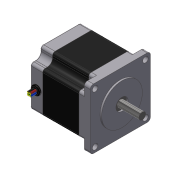
# Autodesk Inventor part: Motor Dummy
Saved by Autodesk Inventor 2015 (Build 190159000, 159)
## iProperties
Created: 2012-06-21
Part Number: Motor Dummy
Material: Generic
Document SubType Name: Modeling
Density: 4.80997 g/cm^3
Categories: <MemberInstance><Categories><Category DisplayName="" Mnemonic="CABLEANDHARNESS" InternalName="e4a7e005-5e42-4d16-b293-125e7f0d0512"><Category DisplayName="" Mnemonic="CONNECTORS" InternalName="6f634eba-a678-4820-a31d-2c2d5ee6728e"><CategoryParameter DisplayName="" Mnemonic="REFDES" InternalName="c3740e8c-60ab-4d5d-8584-52b73222f2f0"/><Category DisplayName="" Mnemonic="DISCRETEWIRE" InternalName="9a3407de-09b2-4cdb-8c40-9708d5144a28"/></Category></Category></Categories><FamilyTemplate><FamilyTemplateParameters></FamilyTemplateParameters></FamilyTemplate><CategoryParameterMap><ParamToTemplateMap><ParamToTemplate CategoryParameter="//CategoryParameter[@InternalName='c3740e8c-60ab-4d5d-8584-52b73222f2f0']" ConstantValue=""/></ParamToTemplateMap></CategoryParameterMap></MemberInstance>
Appearance: Glossy - Black
Mass: 1050 g
Surface Area: 350.377 cm^2
Volume: 218.297 cm^3
Autodesk Inventor part; units mm, degrees
ref_plane "YZ Plane" through (0, 0, 0) normal (1, 0, 0) x (0, 1, 0)
sketch "Sketch1" plane through (0, 0, 0) normal (1, 0, 0) x (0, 1, 0)
  line L0 (-28.2, 28.2) -> (28.2, 28.2)
  line L1 (28.2, 28.2) -> (28.2, -28.2)
  line L2 (28.2, -28.2) -> (-28.2, -28.2)
  line L3 (-28.2, -28.2) -> (-28.2, 28.2)
  point P0 (0, 0)
  point P1 (0, 28.2)
  point P2 (28.2, 0)
  dimension "d0" = 56.4
  dimension "d1" = 56.4
  constraints: 8 end point, 2 midpoint, 2 parallel, 1 horizontal, 1 horizontal alignment, 1 perpendicular, 1 vertical alignment
  measures "d0" distance of L0.start L0.end
  measures "d1" distance of L2.end L0.start
extrude "Extrusion1" add sketch "Sketch1" along normal mid plane 56
hole "Hole1" at (28, 0, 0) direction (-1, 0, 0) diameter 11.5 end through all
sketch "Sketch2" plane through (28, 0, 0) normal (1, 0, 0) x (0, 0, -1)
  line L0 (-23.57, -23.57) -> (23.57, -23.57) construction
  line L1 (23.57, -23.57) -> (23.57, 23.57) construction
  line L2 (23.57, 23.57) -> (-23.57, 23.57) construction
  line L3 (-23.57, 23.57) -> (-23.57, -23.57) construction
  point P0 (0, 0)
  point P1 (0, 23.57)
  point P2 (-23.57, 0)
  dimension "d13" = 47.14
  dimension "d15" = 47.14
  constraints: 8 end point, 4 coincident, 2 midpoint, 2 parallel, 1 horizontal, 1 horizontal alignment, 1 perpendicular, 1 vertical alignment
  measures "d13" distance of L1.end L2.end
  measures "d15" distance of L2.end L0.start
hole "Hole2" at (28, -23.57, 23.57) at (28, 23.57, 23.57) at (28, 23.57, -23.57) at (28, -23.57, -23.57) direction (-1, 0, 0) diameter 5.2 end through all
sketch "Sketch3" plane through (0, 0, 0) normal (0, 1, 0) x (-1, 0, 0)
  line L0 (-28, 28.2) -> (-28, -28.2) projected
  line L1 (73.9, 0) -> (-80.1, 0) projected
  line L2 (-28, 19.05) -> (-29.6, 19.05)
  line L3 (-29.6, 19.05) -> (-29.6, 3.175)
  line L4 (-29.6, 3.175) -> (-48.6, 3.175)
  line L5 (-48.6, 3.175) -> (-48.6, 0)
  line L6 (-28, 19.05) -> (-28, 0)
  line L7 (-29.6, 5.75) -> (-28, 5.75)
  line L8 (-28, 5.75) -> (25, 5.75)
  line L9 (25, 5.75) -> (25, 0)
  line L10 (25, 3.175) -> (42.4, 3.175)
  line L11 (42.4, 3.175) -> (42.4, 0)
  line L12 (28, -28.2) -> (28, 28.2) projected
  line L13 (28, 5.75) -> (-28, 5.75) projected
  line L14 (-29.6, 3.175) -> (-28, 3.175)
  point P0 (0, 0)
  dimension "d23" = 6.35
  dimension "d24" = 38.1
  dimension "d25" = 1.6
  dimension "d26" = 20.6
  dimension "d47" = 6.35
  dimension "d48" = 14.4
  dimension "d49" = 3
  constraints: 22 end point, 9 point on line, 8 perpendicular, 1 collinear, 1 horizontal, 1 midpoint, 1 parallel
  measures "d23" diameter of L4 L1
  measures "d24" diameter of L2 L1
  measures "d25" distance of L2.start L2.end
  measures "d26" distance between parallel lines of L0 L5
  measures "d47" diameter of L10 L1
  measures "d48" distance between parallel lines of L12 L11
  measures "d49" distance between parallel lines of L12 L9
revolve "Revolution1" add sketch "Sketch3" angle 360 about axis through (-10, 0, 0) along (1, 0, 0) contours L0 L7 L3 L2 | L8 L9 L1 L0 | L0 L1 L5 L4 L14 | L10 L12 L1 L9 | L10 L11 L1 L12
sketch "Sketch4" plane through (-28, 0, 0) normal (-1, 0, 0) x (0, 0, 1)
  line L0 (-28.2, 28.2) -> (28.2, 28.2) projected
  line L1 (-28.2, -28.2) -> (-28.2, 28.2) projected
  line L2 (28.2, -28.2) -> (-28.2, -28.2) projected
  line L3 (28.2, 28.2) -> (28.2, -28.2) projected
  line L4 (-28.2, 28.2) -> (-19, 28.2)
  line L5 (-19, 28.2) -> (-19, 19)
  line L6 (-19, 19) -> (-28.2, 19)
  line L7 (-28.2, 19) -> (-28.2, 28.2)
  line L8 (28.2, 28.2) -> (19, 28.2)
  line L9 (19, 28.2) -> (19, 19)
  line L10 (19, 19) -> (28.2, 19)
  line L11 (28.2, 19) -> (28.2, 28.2)
  line L12 (28.2, -28.2) -> (19, -28.2)
  line L13 (19, -28.2) -> (19, -19)
  line L14 (19, -19) -> (28.2, -19)
  line L15 (28.2, -19) -> (28.2, -28.2)
  line L16 (-28.2, -28.2) -> (-19, -28.2)
  line L17 (-19, -28.2) -> (-19, -19)
  line L18 (-19, -19) -> (-28.2, -19)
  line L19 (-28.2, -19) -> (-28.2, -28.2)
  point P0 (0, 0)
  dimension "d28" = 38
  constraints: 32 end point, 8 parallel, 7 equal length, 4 horizontal, 4 perpendicular
  measures "d28" distance between parallel lines of L9 L5
extrude "Extrusion2" cut sketch "Sketch4" against normal blind 50.5 contours L0 L5 L6 L1 | L0 L3 L10 L9 | L18 L17 L2 L1 | L3 L2 L13 L14
fillet "Fillet1" radius 2.3 8 edges at (-2.75, -19, 28.2) (-2.75, -28.2, 19) (-2.75, -28.2, -19) (-2.75, -19, -28.2) (-2.75, 19, -28.2) (-2.75, 28.2, -19) (-2.75, 28.2, 19) (-2.75, 19, 28.2)
fillet "Fillet1" radius 5 4 edges at (-2.75, -19, 19) (-2.75, 19, 19) (-2.75, 19, -19) (-2.75, -19, -19)
fillet "Fillet1" radius 3 4 edges at (25.25, -28.2, 28.2) (25.25, -28.2, -28.2) (25.25, 28.2, 28.2) (25.25, 28.2, -28.2)
fillet "Fillet2" radius 1 24 edges at (-28, -18.3263, 27.5263) (-28, -19, 24.95) (-28, -20.4645, 20.4645) (-28, -24.95, 19) (-28, -27.5263, 18.3263) (-28, -28.2, 0) (-28, -27.5263, -18.3263) (-28, -24.95, -19) (-28, -20.4645, -20.4645) (-28, -19, -24.95) (-28, -18.3263, -27.5263) (-28, 0, -28.2) (-28, 18.3263, -27.5263) (-28, 19, -24.95) (-28, 20.4645, -20.4645) (-28, 24.95, -19) (-28, 27.5263, -18.3263) (-28, 28.2, 0) (-28, 27.5263, 18.3263) (-28, 24.95, 19) (-28, 20.4645, 20.4645) (-28, 19, 24.95) (-28, 18.3263, 27.5263) (-28, 0, 28.2)
ref_plane "Work Plane1" through (17.5, 0, 0) normal (1, 0, 0) x (0, 0, -1)
ref_plane "Work Plane2" through (-16.5, 0, 0) normal (-1, 0, 0) x (0, 0, 1)
split body "Split1" result two bodies by plane through (-16.5, 0, 0) normal (-1, 0, 0) first body at (-17, 6.6969, -6.433)
split body "Split2" result two bodies by plane through (17.5, 0, 0) normal (1, 0, 0) bodies 3 first body at (18, -6.6969, -6.9609)
sketch "Sketch5" plane through (-27, -28.2, -16.7) normal (0, -1, 0) x (1, 0, 0)
  circle A0 centre (5, 16.7) radius 4.25
  line L0 (-1, 33.4) -> (-1, 0) projected
  point P0 (27, 16.7)
  dimension "d37" = 8.5
  dimension "d38" = 6
  constraints: 1 centre point, 1 horizontal alignment
  measures "d37" diameter of A0
  measures "d38" distance from line of L0 A0.centre
extrude "Extrusion3" add sketch "Sketch5" along normal mid plane 4 bodies 2
sketch "Sketch6" plane through (-22, -30.2, 0) normal (0, -1, 0) x (1, 0, 0)
  circle A0 centre (-1, 1) radius 1
  circle A1 centre (1, 1) radius 1
  circle A2 centre (1, -1) radius 1
  circle A3 centre (-1, -1) radius 1
  circle A4 centre (0, 0) radius 4.25 projected
  point P0 (22, 0)
  dimension "d41" = 2
  dimension "d42" = 1
  dimension "d43" = 1
  constraints: 7 equal radius, 4 centre point, 1 horizontal alignment, 1 vertical alignment
  measures "d41" diameter of A0
  measures "d42" horizontal distance of A4.centre A0.centre
  measures "d43" horizontal distance of A4.centre A0.centre
extrude "Extrusion4" add sketch "Sketch6" along normal blind 5 contours A0 | A1 | A3 | A2 bodies 2
fillet "Fillet3" radius 1 1 edges at (-26.25, -30.2, 0)
sketch "Sketch7" plane through (-22, -35.2, 0) normal (0, -1, 0) x (1, 0, 0)
  arc A0 (-1, 0) -> (0, -1) centre (-1, -1) ccw projected
sketch "Sketch8" plane through (-22, -35.2, 0) normal (0, -1, 0) x (1, 0, 0)
  arc A0 (0, 1) -> (-1, 0) centre (-1, 1) ccw projected
sketch "Sketch9" plane through (-22, -35.2, 0) normal (0, -1, 0) x (1, 0, 0)
  arc A0 (1, 0) -> (0, -1) centre (1, -1) ccw projected
sketch "Sketch10" plane through (-22, -35.2, 0) normal (0, -1, 0) x (1, 0, 0)
  arc A0 (1, 0) -> (0, 1) centre (1, 1) ccw projected
equation "\"d4\" = 0.5 * d1"
equation "\"d14\" = 0.5 * d1"
equation "\"d15\" = d13"
equation "\"d47\" = d23"
body "Solid2"
body "Solid4"
body "Solid5"
